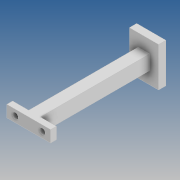
# Autodesk Inventor part: LickModuleMount_Lobster
Saved by Autodesk Inventor 2020 (Build 240168000, 168)
## iProperties
Created: 2019-08-06
Part Number: LickModuleMount_Lobster
Material: 일반
Document SubType Name: Modeling
Designer: Jeong Ji Hoon
Density: 1 g/cm^3
Appearance: 기본값
Author: Jeong Ji Hoon
## iProperties of the stored document _3D 인쇄.ipt
Created: 2019-08-06
Part Number: _3D 인쇄
Material: 일반
Document SubType Name: Modeling
Designer: Jeong Ji Hoon
Density: 1 g/cm^3
Appearance: 기본값
Author: Jeong Ji Hoon
Autodesk Inventor part; units mm, degrees
ref_plane "YZ Plane" through (0, 0, 0) normal (1, 0, 0) x (0, 1, 0)
ref_plane "XZ Plane" through (0, 0, 0) normal (0, 1, 0) x (-1, 0, 0)
ref_plane "XY Plane" through (0, 0, 0) normal (0, 0, 1) x (1, 0, 0)
sketch "스케치1" plane through (0, 0, 0) normal (0, 0, 1) x (1, 0, 0)
  line L0 (0, 0) -> (20, 0)
  line L1 (20, 0) -> (20, 27)
  line L2 (20, 27) -> (0, 27)
  line L3 (0, 27) -> (0, 0)
  dimension "d0" = 20
  dimension "d1" = 27
  constraints: 8 end point, 2 parallel, 1 horizontal, 1 perpendicular
  measures "d0" distance of L2.end L1.end
  measures "d1" distance of L1.end L0.end
extrude "돌출1" add sketch "스케치1" along normal blind 5
sketch "스케치2" plane through (0, 0, 5) normal (0, 0, 1) x (1, 0, 0)
  line L0 (0, 27) -> (0, 0) projected
  line L1 (20, 27) -> (0, 27) projected
  line L2 (6, 18.5) -> (14, 18.5)
  line L3 (14, 18.5) -> (14, 8.5)
  line L4 (14, 8.5) -> (6, 8.5)
  line L5 (6, 8.5) -> (6, 18.5)
  point P0 (6, 13.5)
  point P1 (0, 13.5)
  point P2 (10, 18.5)
  point P3 (10, 27)
  dimension "d4" = 8
  dimension "d5" = 10
  constraints: 8 end point, 4 midpoint, 2 parallel, 1 horizontal, 1 horizontal alignment, 1 perpendicular, 1 vertical alignment
  measures "d4" distance of L3.end L4.end
  measures "d5" distance of L2.end L3.end
extrude "돌출2" add sketch "스케치2" along normal blind 75
sketch "스케치3" plane through (0, 0, 80) normal (0, 0, 1) x (1, 0, 0)
  line L0 (14, 18.5) -> (6, 18.5) projected
  line L1 (-5, 18.5) -> (25, 18.5)
  line L2 (25, 18.5) -> (25, 10.5)
  line L3 (25, 10.5) -> (-5, 10.5)
  line L4 (-5, 10.5) -> (-5, 18.5)
  point P0 (0, 0)
  point P1 (10, 18.5)
  point P2 (10, 10.5)
  dimension "d8" = 30
  dimension "d42" = 8
  constraints: 8 end point, 3 midpoint, 2 parallel, 1 horizontal, 1 perpendicular
  measures "d8" distance of L1.start L1.end
  measures "d42" distance of L1.end L2.end
extrude "돌출11" add sketch "스케치3" along normal blind 4
sketch "스케치9" plane through (0, 0, 84) normal (0, 0, 1) x (1, 0, 0)
  line L0 (25, 10.5) -> (25, 18.5) projected
  line L1 (25, 18.5) -> (-5, 18.5) projected
  line L2 (-5, 18.5) -> (-5, 10.5) projected
  point P0 (0, 0)
  point P1 (0.75, 14.5)
  point P2 (19.25, 14.5)
  dimension "d45" = 4
  dimension "d46" = 5.75
  dimension "d47" = 5.75
  measures "d45" distance from line of L1 point (0.75, 14.5)
  measures "d46" distance from line of L2 point (0.75, 14.5)
  measures "d47" distance from line of L0 point (19.25, 14.5)
hole "구멍2" at (0.75, 14.5, 84) at (19.25, 14.5, 84) direction (0, 0, -1) diameter 4 depth 4 tip angle 118
sketch "스케치10" plane through (6, 8.5, 5) normal (-1, 0, 0) x (0, 0, 1)
  line L0 (50.5712, 8.6876) -> (57.0225, 8.6876) construction
  line L1 (57.0225, 8.6876) -> (57.0225, 1.7484) construction
  line L2 (57.0225, 1.7484) -> (50.5712, 1.7484) construction
  line L3 (50.5712, 1.7484) -> (50.5712, 8.6876) construction
  spline S0 degree 2 poles (54.4395, 7.018) (54.1199, 6.6323) (53.4917, 6.3568) knots 0 0 0 1 1 1
  line L4 (53.4917, 6.3568) -> (53.1996, 6.9519)
  spline S1 degree 2 poles (53.1996, 6.9519) (53.7837, 7.1833) (54.5221, 8.1972) (54.5221, 8.6876) knots 0 0 0 1 2 2 2
  line L5 (54.5221, 8.6876) -> (55.1062, 8.6876)
  spline S2 degree 2 poles (55.1062, 8.6876) (55.1062, 8.1917) (55.8556, 7.1778) (56.4287, 6.9519) knots 0 0 0 1 2 2 2
  line L6 (56.4287, 6.9519) -> (56.1367, 6.3568)
  spline S3 degree 2 poles (56.1367, 6.3568) (55.6022, 6.5992) (55.1889, 7.0235) knots 0 0 0 1 1 1
  line L7 (55.1889, 7.0235) -> (55.1889, 1.8327)
  line L8 (55.1889, 1.8327) -> (54.4395, 1.8327)
  line L9 (54.4395, 1.8327) -> (54.4395, 7.018)
  point P0 (-5, -8.5)
  constraints: 2 other
extrude "돌출12" add sketch "스케치10" along normal blind 1
